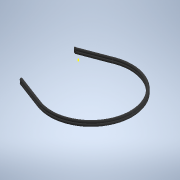
# Autodesk Inventor part: Oring 2-161 Deform
Saved by Autodesk Inventor 2020.3 (Build 243373000, 373)
## iProperties
Created: 2020-07-05
Part Number: Oring 2-161 Deform
Material: Rubber
Document SubType Name: Modeling
Designer: Bruno
Density: 0.93 g/cm^3
Appearance: Rubber - Black
Author: Bruno
Autodesk Inventor part; units mm, degrees
ref_plane "YZ Plane" through (0, 0, 0) normal (1, 0, 0) x (0, 1, 0)
ref_plane "Work Plane1" through (0, 1.343, 0) normal (0, 1, 0) x (-1, 0, 0)
sketch "Sketch1" plane through (0, 0, 0) normal (1, 0, 0) x (0, 1, 0)
  point P0 (0, 0)
sketch "Sketch2" plane through (0, 1.343, 0) normal (0, 1, 0) x (-1, 0, 0)
  point P0 (0, 0)
ref_plane "Work Plane2" through (18.5889, -0.0573, 58.9222) normal (0.9356, 0, 0.3531) x (0, 1, 0)
sketch "Sketch3" plane through (18.5889, -0.0573, 58.9222) normal (0.9356, 0, 0.3531) x (0, 1, 0)
  circle A0 centre (0, 0) radius 1.3
  point P0 (0.0573, -48.561)
  dimension "d19" = 2.6
  constraints: 1 centre point
  measures "d19" diameter of A0
sketch3d "3D Sketch1"
  line L0 (-8.9168, -0.0573, 48.5396) -> (18.5889, -0.0573, 58.9222)
  arc A0 (18.5889, -0.0573, 58.9222) -> (74.9435, -0.0573, 21.0473) centre (34.0387, -0.0573, 21.0473) ccw
  arc A1 (74.9435, -0.0573, 21.0473) -> (18.5889, -0.0432, -16.8275) centre (34.0387, -0.0573, 21.0473) ccw
  line L1 (18.5889, -0.0432, -16.8275) -> (-8.9168, -0.0437, -6.445)
  dimension "d0" = 2.8
  dimension "d1" = 51
  dimension "d9" = 29.4
  dimension "d12" = 51
  dimension "d14" = 29.4
  dimension "d16" = 2.8
  dimension "d17" = 1.343
  dimension "d18" = -0.057
sweep "Sweep1" add profiles "Sketch3" path "3D Sketch1"
ref_plane "Work Plane3" through (18.5889, 2.7292, -16.8275) normal (0.9356, 0, -0.3531) x (0, 1, 0)
sketch "Sketch4" plane through (18.5889, 2.7292, -16.8275) normal (0.9356, 0, -0.3531) x (0, 1, 0)
  circle A0 centre (0, 0) radius 1.3
  point P0 (-2.7295, 9.1787)
  dimension "d22" = 2.6
  constraints: 1 centre point
  measures "d22" diameter of A0
sketch3d "3D Sketch1 for Sweep2"
  line L0 (-8.9168, -0.0703, -6.445) -> (-8.9168, 2.7297, -6.445)
  line L1 (-8.9168, 2.7297, -6.445) -> (18.5889, 2.7292, -16.8275)
  arc A0 (18.5889, 2.7292, -16.8275) -> (74.9435, 2.7433, 21.0473) centre (34.0387, 2.7433, 21.0473) ccw
  arc A1 (74.9435, 2.7433, 21.0473) -> (18.5889, 2.7433, 58.9222) centre (34.0387, 2.7433, 21.0473) ccw
  line L2 (18.5889, 2.7433, 58.9222) -> (-8.9168, 2.7433, 48.5396)
  line L3 (-8.9168, 2.7433, 48.5396) -> (-8.9168, -0.0567, 48.5396)
  dimension "d0" = 2.8
  dimension "d1" = 51
  dimension "d9" = 29.4
  dimension "d12" = 51
  dimension "d14" = 29.4
  dimension "d16" = 2.8
  dimension "d17" = 1.343
  dimension "d18" = -0.057
sweep "Sweep2" add profiles "Sketch4" path "3D Sketch1 for Sweep2" separate body
sketch "Sketch5" plane through (0, 1.343, 0) normal (0, 1, 0) x (-1, 0, 0)
  ellipse E0 centre (-18.5889, -16.8275) end of major axis (-18.0979, -18.0312) minor radius 0.0002 (-18.5868, -16.8332) -> (-18.5889, -16.827) ccw projected
  circle A0 centre (-34.0404, 21.0517) radius 40.909
  point P0 (0, 0)
  constraints: 4 other
body "Solid1"
body "Solid2"
